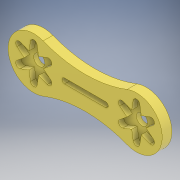
# Autodesk Inventor part: Pata - Antebrazo
Saved by Autodesk Inventor 2019 (Build 230136000, 136)
## iProperties
Created: 2020-02-11
Part Number: Pata - Antebrazo
Material: ABS Plastic
Document SubType Name: Modeling
Designer: jacqu
Density: 1.06 g/cm^3
Appearance: Smooth - White
Mass: 6.28509 g
Surface Area: 55.6042 cm^2
Volume: 5.92933 cm^3
d0: 20.000 mm
diametro_petalo: 2.600 mm
diametro_aspa: 14.900 mm
largo_petalo: 7.300 mm
Author: jacqu
Autodesk Inventor part; units mm, degrees
ref_plane "YZ Plane" through (0, 0, 0) normal (1, 0, 0) x (0, 1, 0)
ref_plane "XZ Plane" through (0, 0, 0) normal (0, 1, 0) x (-1, 0, 0)
sketch "Sketch1" plane through (0, 0, 0) normal (0, 0, 1) x (1, 0, 0)
  arc A0 (-72.7273, 18.6308) -> (-72.7273, -18.6308) centre (-80, 0) ccw
  arc A1 (-7.2727, -18.6308) -> (-72.7273, -18.6308) centre (-40, -102.4695) ccw
  arc A2 (-7.2727, -18.6308) -> (-7.2727, 18.6308) centre (0, 0) ccw
  arc A3 (-72.7273, 18.6308) -> (-7.2727, 18.6308) centre (-40, 102.4695) ccw
  arc A4 (-79.5765, 3.9775) -> (-79.5765, -3.9775) centre (-80, 0) ccw
  arc A5 (-0.4235, -3.9775) -> (-0.4235, 3.9775) centre (0, 0) ccw
  arc A6 (-80.4235, -3.9775) -> (-80.4235, 3.9775) centre (-80, 0) ccw
  arc A7 (-0.4235, 3.9775) -> (-0.4235, -3.9775) centre (0, 0) ccw
  point P0 (-103.8261, -115.9088)
  dimension "d0" = 20
  dimension "d1" = 20
  dimension "d2" = 90
  dimension "d3" = 90
  dimension "d4" = 4
  dimension "d7" = 80
  dimension "d33" = 4
  constraints: 18 point on circle, 8 centre point, 6 tangent, 3 coincident, 2 equal radius, 1 horizontal alignment
  measures "d0" radius of A0
  measures "d1" radius of A2
  measures "d2" radius of A3
  measures "d3" radius of A1
  measures "d4" radius of A4
  measures "d7" distance of A5.centre A4.centre
  measures "d33" radius of A6
extrude "Extrusion1" add sketch "Sketch1" along normal blind 7.55 contours A3 A2 A1 A0 | A6 A4 | A7 A5
sketch "Sketch3" plane through (0, 0, 7.55) normal (0, 0, 1) x (1, 0, 0)
  arc A0 (-72.7273, 18.6308) -> (-72.7273, -18.6308) centre (-80, 0) ccw projected
  arc A1 (-7.2727, -18.6308) -> (-72.7273, -18.6308) centre (-40, -102.4695) ccw projected
  arc A2 (-7.2727, -18.6308) -> (-7.2727, 18.6308) centre (0, 0) ccw projected
  arc A3 (-72.7273, 18.6308) -> (-7.2727, 18.6308) centre (-40, 102.4695) ccw projected
  line L0 (-56.02, 2) -> (-23.98, 2)
  line L1 (-56.02, -2) -> (-23.98, -2)
  arc A4 (-56.02, 2) -> (-56.02, -2) centre (-56.02, 0) ccw
  arc A5 (-23.98, -2) -> (-23.98, 2) centre (-23.98, 0) ccw
  point P0 (-83.48, 0)
  dimension "d12" = 2
  constraints: 4 end point, 4 point on circle, 4 tangent, 2 centre point, 2 horizontal, 1 horizontal alignment
  measures "d12" radius of A4
extrude "Extrusion2" cut sketch "Sketch3" against normal blind 10 contours L0 A5 L1 A4
ref_plane "Work Plane2" through (-40, 0, 7.55) normal (-1, 0, 0) x (0, -1, 0)
ref_plane "Work Plane1" through (-100, 0, 7.55) normal (-1, 0, 0) x (0, -1, 0)
sketch "Sketch10" plane through (0, 0, 0) normal (0, 0, -1) x (-1, 0, 0)
  circle A0 centre (0, 0) radius 4.35
  dimension "d43" = 8.7
  constraints: 1 centre point, 1 coincident
  measures "d43" diameter of A0
extrude "Extrusion7" cut sketch "Sketch10" against normal blind 10
mirror "Mirror4" about plane through (-40, 0, 7.55) normal (-1, 0, 0) of "Extrusion7"
sketch "Sketch9" plane through (0, 0, 0) normal (0, 0, -1) x (-1, 0, 0)
  arc A0 (13.113, 4.6066) -> (10.5459, 9.0529) centre (11.4723, 6.6235) ccw
  arc A1 (2.5671, 13.6595) -> (-2.5671, 13.6595) centre (0, 13.2471) ccw
  line L0 (13.113, 4.6066) -> (7.45, 0)
  line L1 (10.5459, 9.0529) -> (3.725, 6.4519)
  line L2 (3.725, 6.4519) -> (2.5671, 13.6595)
  line L3 (-2.5671, 13.6595) -> (-3.725, 6.4519)
  line L4 (-3.725, 6.4519) -> (-10.5459, 9.0529)
  line L5 (-13.113, 4.6066) -> (-7.45, 0)
  arc A2 (-10.5459, 9.0529) -> (-13.113, 4.6066) centre (-11.4723, 6.6235) ccw
  arc A3 (72.7273, -18.6308) -> (72.7273, 18.6308) centre (80, 0) ccw projected
  arc A4 (7.2727, 18.6308) -> (72.7273, 18.6308) centre (40, 102.4695) ccw projected
  arc A5 (7.2727, 18.6308) -> (7.2727, -18.6308) centre (0, 0) ccw projected
  arc A6 (72.7273, -18.6308) -> (7.2727, -18.6308) centre (40, -102.4695) ccw projected
  circle A7 centre (0, 0) radius 7.45 construction
  line L6 (-7.45, 0) -> (7.45, 0) construction
  arc A8 (10.5459, -9.0529) -> (13.113, -4.6066) centre (11.4723, -6.6235) ccw
  arc A9 (-2.5671, -13.6595) -> (2.5671, -13.6595) centre (0, -13.2471) ccw
  line L7 (13.113, -4.6066) -> (7.45, 0)
  line L8 (10.5459, -9.0529) -> (3.725, -6.4519)
  line L9 (3.725, -6.4519) -> (2.5671, -13.6595)
  line L10 (-2.5671, -13.6595) -> (-3.725, -6.4519)
  line L11 (-3.725, -6.4519) -> (-10.5459, -9.0529)
  line L12 (-13.113, -4.6066) -> (-7.45, 0)
  arc A10 (-13.113, -4.6066) -> (-10.5459, -9.0529) centre (-11.4723, -6.6235) ccw
  circle A11 centre (0, 0) radius 4.35
  dimension "diametro_petalo" = 2.6
  dimension "diametro_aspa" = 14.9
  dimension "largo_petalo" = 7.3
  dimension "d52" = 60
  dimension "d53" = 8.7
  constraints: 26 end point, 18 point on circle, 11 symmetric about line, 8 centre point, 5 equal length, 5 tangent, 3 coincident, 3 horizontal alignment, 2 equal radius, 1 vertical alignment, 3 other
  measures "diametro_petalo" radius of A0
  measures "diametro_aspa" diameter of A7
  measures "largo_petalo" distance of L0.start L0.end
  measures "d53" diameter of A11
extrude "Extrusion8" cut sketch "Sketch9" against normal blind 4.25 contours L0 L7 A8 L8 L9 A9 L10 L11 A10 L12 L5 A2 L4 L3 A1 L2 L1 A0
mirror "Mirror5" about plane through (-40, 0, 7.55) normal (-1, 0, 0) of "Extrusion8"
equation "\"d0\" = radio_muslo"
equation "\"d1\" = d0"
equation "\"d2\" = curva"
equation "\"d3\" = d2"
equation "\"d4\" = 0.5 * diametro_servo"
equation "\"d7\" = distancia_centros"
equation "\"d33\" = d4"
equation "\"curva\" = 90"
equation "\"distancia_centros\" = 80"
equation "\"espesor\" = 3.3"
equation "\"diametro_servo\" = 8"
equation "\"radio_muslo\" = 20"
body "Solid1"
